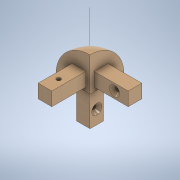
# Autodesk Inventor part: ZakulacenaCast
Saved by Autodesk Inventor 2022 (Build 260153000, 153)
## iProperties
Created: 2021-05-12
Part Number: ZakulacenaCast
Material: Všeobecné
Document SubType Name: Modeling
Designer: peepu
Density: 1 g/cm^3
Appearance: Strakatá
Author: peepu
Autodesk Inventor part; units mm, degrees
ref_plane "YZ Plane" through (0, 0, 0) normal (1, 0, 0) x (0, 1, 0)
ref_plane "XZ Plane" through (0, 0, 0) normal (0, 1, 0) x (-1, 0, 0)
ref_plane "XY Plane" through (0, 0, 0) normal (0, 0, 1) x (1, 0, 0)
sketch "Náčrt1" plane through (0, 0, 0) normal (1, 0, 0) x (0, 1, 0)
  line L0 (0, 0) -> (50, 0)
  line L1 (50, 0) -> (50, -50)
  line L2 (50, -50) -> (0, -50)
  line L3 (0, -50) -> (0, 0)
  arc A0 (0, -50) -> (50, 0) centre (0, 0) ccw
  line L4 (0, 0) -> (6, 0)
  line L5 (0, -6) -> (0, 0)
  line L6 (6, -6) -> (26, -6)
  line L7 (26, -6) -> (26, -26)
  line L8 (26, -26) -> (6, -26)
  line L9 (6, -26) -> (6, -6)
  dimension "d0" = 50
  dimension "d1" = 50
  dimension "d2" = 50
  dimension "d4" = 6
  dimension "d5" = 6
  dimension "d6" = 20
  dimension "d7" = 20
  constraints: 20 end point, 4 parallel, 3 horizontal, 2 perpendicular, 2 point on circle, 1 centre point
  measures "d0" distance of L1.end L2.end
  measures "d1" distance of L0.end L1.end
  measures "d2" radius of A0
  measures "d4" distance of L6.start L5.start
  measures "d5" distance of L4.end L6.start
  measures "d6" distance of L7.end L8.end
  measures "d7" distance of L6.end L7.end
extrude "Vysunutí1" add sketch "Náčrt1" against normal blind 50 contours L0 A0 L3 | L1 L2 A0 | L6 L7 L8 L9
revolve "Rotace1" cut sketch "Náčrt1" angle 90 about axis through (0, 0, 0) along (0, 1, 0) keep common part contours L0 A0 L3 | L6 L7 L8 L9
extrude "Vysunutí2" add sketch "Náčrt1" along normal blind 50 contours L6 L7 L8 L9
sketch "Náčrt2" plane through (0, 6, -6) normal (0, 0, 1) x (1, 0, 0)
  line L0 (50, 20) -> (50, 0) projected
  line L1 (0, 0) -> (50, 0) projected
  point P0 (0, -6)
  point P1 (30, 10)
  dimension "d13" = 20
  dimension "d21" = 10
  measures "d13" distance from line of L0 point (30, 10)
  measures "d21" distance from line of L1 point (30, 10)
hole "Díra1" at (30, 16, -6) direction (0, 0, -1) diameter 6 end through all countersink diameter 15 countersink angle 90
pattern_circular "Kruhové pole1" count 3 over 360 about axis through (0, 0, 0) along (-0.5774, 0.5774, -0.5774) of "Vysunutí2", "Díra1"
